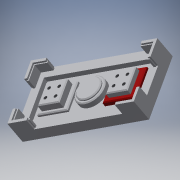
# Autodesk Inventor part: batteryCellTop
Saved by Autodesk Inventor 2019 (Build 230136000, 136)
## iProperties
Created: 2013-02-12
Part Number: batteryCellTop
Material: Aluminum 6061
Document SubType Name: Modeling
Designer: user
Density: 2.71 g/cm^3
Mass: 246.958 g
Surface Area: 283.047 cm^2
Volume: 91.1285 cm^3
Appearance: Aluminum - Flat
Description: BattTop
Author: user
Revision Number: 1
Autodesk Inventor part; units mm, degrees
ref_plane "YZ Plane" through (0, 0, 0) normal (1, 0, 0) x (0, 1, 0)
ref_plane "XZ Plane" through (0, 0, 0) normal (0, 1, 0) x (-1, 0, 0)
ref_plane "XY Plane" through (0, 0, 0) normal (0, 0, 1) x (1, 0, 0)
sketch "Sketch1" plane through (0, 0, 0) normal (0, 1, 0) x (-1, 0, 0)
  line L0 (62.25, -32.4) -> (-62.25, -32.4)
  line L1 (-62.25, -32.4) -> (-62.25, 32.4)
  line L2 (-62.25, 32.4) -> (62.25, 32.4)
  line L3 (62.25, 32.4) -> (62.25, -32.4)
  point P0 (0, 0)
  point P1 (62.25, 0)
  point P2 (0, -32.4)
  dimension "d0" = 64.8
  dimension "d2" = 124.5
  constraints: 8 end point, 2 midpoint, 2 parallel, 1 horizontal, 1 horizontal alignment, 1 perpendicular, 1 vertical alignment
  measures "d0" distance of L2.end L0.start
  measures "d2" distance of L0.start L0.end
extrude "Extrusion1" add sketch "Sketch1" along normal blind 11.45
sketch "Sketch2" plane through (0, 11.45, 0) normal (0, 1, 0) x (1, 0, 0)
  line L0 (62.25, 32.4) -> (-62.25, 32.4) projected
  line L1 (-62.25, 32.4) -> (-62.25, -32.4) projected
  line L2 (-62.25, -32.4) -> (62.25, -32.4) projected
  line L3 (62.25, -32.4) -> (62.25, 32.4) projected
  line L4 (-62.25, -13.55) -> (-62.25, -32.4)
  line L5 (-62.25, -32.4) -> (-46.85, -32.4)
  line L6 (-46.85, -32.4) -> (-46.85, -29.5)
  line L7 (-46.85, -29.5) -> (-59.35, -29.5)
  line L8 (-59.35, -29.5) -> (-59.35, -13.55)
  line L9 (-59.35, -13.55) -> (-62.25, -13.55)
  line L10 (62.25, -13.55) -> (59.35, -13.55)
  line L11 (59.35, -13.55) -> (59.35, -29.5)
  line L12 (59.35, -29.5) -> (46.85, -29.5)
  line L13 (46.85, -29.5) -> (46.85, -32.4)
  line L14 (62.25, -32.4) -> (62.25, -13.55)
  line L15 (46.85, -32.4) -> (62.25, -32.4)
  line L16 (43.4, 32.4) -> (43.4, 29.5)
  line L17 (43.4, 29.5) -> (59.35, 29.5)
  line L18 (62.25, 32.4) -> (43.4, 32.4)
  line L19 (59.35, 29.5) -> (59.35, 17)
  line L20 (59.35, 17) -> (62.25, 17)
  line L21 (62.25, 17) -> (62.25, 32.4)
  line L22 (-62.25, 17) -> (-59.35, 17)
  line L23 (-59.35, 17) -> (-59.35, 29.5)
  line L24 (-59.35, 29.5) -> (-43.4, 29.5)
  line L25 (-43.4, 29.5) -> (-43.4, 32.4)
  line L26 (-62.25, 32.4) -> (-62.25, 17)
  line L27 (-43.4, 32.4) -> (-62.25, 32.4)
  point P0 (0, 0)
  dimension "d5" = 18.85
  dimension "d7" = 15.4
  dimension "d8" = 2.9
  dimension "d9" = 2.9
  dimension "d10" = 18.85
  dimension "d11" = 2.9
  dimension "d12" = 2.9
  dimension "d13" = 15.4
  dimension "d21" = 15.4
  dimension "d22" = 18.85
  dimension "d23" = 2.9
  dimension "d24" = 2.9
  dimension "d28" = 15.4
  dimension "d29" = 2.9
  dimension "d30" = 2.9
  dimension "d31" = 18.85
  constraints: 48 end point, 13 parallel, 9 perpendicular, 6 collinear, 2 point on line
  measures "d5" distance between parallel lines of L5 L9
  measures "d7" distance of L4.end L5.end
  measures "d8" distance between parallel lines of L8 L4
  measures "d9" distance between parallel lines of L5 L7
  measures "d10" distance of L2.end L10.start
  measures "d11" distance of L10.start L10.end
  measures "d12" distance of L12.end L13.end
  measures "d13" distance of L13.end L2.end
  measures "d21" distance between parallel lines of L18 L20
  measures "d22" distance of L18.start L18.end
  measures "d23" distance between parallel lines of L19 L21
  measures "d24" distance between parallel lines of L18 L17
  measures "d28" distance of L27.end L26.end
  measures "d29" distance of L26.end L23.start
  measures "d30" distance of L24.end L27.start
  measures "d31" distance of L27.start L27.end
extrude "Extrusion2" add sketch "Sketch2" along normal blind 11.3 contours L3 L20 L19 L17 L16 L0 | L25 L24 L23 L22 L1 L0 | L3 L2 L13 L12 L11 L10 | L9 L8 L7 L6 L2 L1
sketch "Sketch3" plane through (0, 11.45, 0) normal (0, 1, 0) x (1, 0, 0)
  line L0 (43.4, 32.4) -> (-43.4, 32.4) projected
  line L1 (-62.25, 17) -> (-62.25, -13.55) projected
  line L2 (-46.85, -32.4) -> (46.85, -32.4) projected
  line L3 (62.25, -13.55) -> (62.25, 17) projected
  line L4 (-53.25, 22.4) -> (53.25, 22.4)
  line L5 (53.25, 22.4) -> (53.25, -22.4)
  line L6 (53.25, -22.4) -> (-53.25, -22.4)
  line L7 (-53.25, -22.4) -> (-53.25, 22.4)
  point P0 (0, 0)
  dimension "d41" = 9
  dimension "d42" = 9
  dimension "d43" = 10
  dimension "d44" = 10
  constraints: 8 end point, 2 parallel, 1 horizontal, 1 perpendicular
  measures "d41" distance between parallel lines of L1 L7
  measures "d42" distance between parallel lines of L3 L5
  measures "d43" distance between parallel lines of L4 L0
  measures "d44" distance between parallel lines of L2 L6
extrude "Extrusion3" cut sketch "Sketch3" against normal blind 5.1
sketch "Sketch4" plane through (0, 6.35, 0) normal (0, 1, 0) x (1, 0, 0)
  line L0 (-53.25, -22.4) -> (-53.25, 22.4) projected
  line L1 (-49.65, 15.75) -> (-17.15, 15.75)
  line L2 (-17.15, 15.75) -> (-17.15, -15.75)
  line L3 (-17.15, -15.75) -> (-49.65, -15.75)
  line L4 (-49.65, -15.75) -> (-49.65, 15.75)
  line L5 (43.4, 32.4) -> (-43.4, 32.4) projected
  point P0 (0, 0)
  dimension "d47" = 32.5
  dimension "d49" = 31.5
  dimension "d50" = 16.65
  dimension "d51" = 3.6
  constraints: 8 end point, 2 parallel, 1 horizontal, 1 perpendicular
  measures "d47" distance between parallel lines of L2 L4
  measures "d49" distance between parallel lines of L3 L1
  measures "d50" distance between parallel lines of L1 L5
  measures "d51" distance between parallel lines of L4 L0
extrude "Extrusion4" add sketch "Sketch4" along normal blind 4.6
sketch "Sketch5" plane through (0, 10.95, 0) normal (0, 1, 0) x (1, 0, 0)
  line L0 (-17.15, 15.75) -> (-49.65, 15.75) projected
  line L1 (-49.65, 15.75) -> (-49.65, -15.75) projected
  line L2 (-44.1, 11.95) -> (-22.7, 11.95)
  line L3 (-22.7, 11.95) -> (-22.7, -11.95)
  line L4 (-22.7, -11.95) -> (-44.1, -11.95)
  line L5 (-44.1, -11.95) -> (-44.1, 11.95)
  point P0 (0, 0)
  point P1 (-33.4, 11.95)
  point P2 (-33.4, 15.75)
  point P3 (-44.1, 0)
  point P4 (-49.65, 0)
  dimension "d54" = 21.4
  dimension "d56" = 23.9
  constraints: 8 end point, 4 midpoint, 2 parallel, 1 horizontal, 1 horizontal alignment, 1 perpendicular, 1 vertical alignment
  measures "d54" distance of L2.start L2.end
  measures "d56" distance between parallel lines of L4 L2
extrude "Extrusion5" add sketch "Sketch5" along normal blind 5.5
sketch "Sketch6" plane through (0, 6.35, 0) normal (0, 1, 0) x (1, 0, 0)
  line L0 (53.25, 22.4) -> (53.25, -22.4) projected
  line L1 (18.73, 14.8) -> (48.73, 14.8)
  line L2 (48.73, 14.8) -> (48.73, -14.8)
  line L3 (48.73, -14.8) -> (18.73, -14.8)
  line L4 (18.73, -14.8) -> (18.73, 14.8)
  point P0 (0, 0)
  point P1 (18.73, 0)
  dimension "d59" = 29.6
  dimension "d61" = 30
  dimension "d62" = 4.52
  constraints: 8 end point, 2 parallel, 1 horizontal, 1 horizontal alignment, 1 midpoint, 1 perpendicular
  measures "d59" distance between parallel lines of L3 L1
  measures "d61" distance of L1.start L1.end
  measures "d62" distance between parallel lines of L0 L2
extrude "Extrusion6" add sketch "Sketch6" along normal blind 2.8
sketch "Sketch7" plane through (0, 9.15, 0) normal (0, 1, 0) x (1, 0, 0)
  line L0 (48.73, 14.8) -> (18.73, 14.8) projected
  line L1 (18.73, 14.8) -> (18.73, -14.8) projected
  line L2 (23.03, 11.95) -> (44.43, 11.95)
  line L3 (44.43, 11.95) -> (44.43, -11.95)
  line L4 (44.43, -11.95) -> (23.03, -11.95)
  line L5 (23.03, -11.95) -> (23.03, 11.95)
  point P0 (0, 0)
  point P1 (23.03, 0)
  point P2 (18.73, 0)
  point P3 (33.73, 11.95)
  point P4 (33.73, 14.8)
  dimension "d65" = 21.4
  dimension "d67" = 23.9
  constraints: 8 end point, 4 midpoint, 2 parallel, 1 horizontal, 1 horizontal alignment, 1 perpendicular, 1 vertical alignment
  measures "d65" distance of L2.start L2.end
  measures "d67" distance of L2.end L3.end
extrude "Extrusion7" add sketch "Sketch7" along normal blind 7.3
sketch "Sketch8" plane through (0, 11.45, 0) normal (0, 1, 0) x (1, 0, 0)
  line L0 (62.25, -13.55) -> (62.25, 17) projected
  line L1 (-60.55, -12.55) -> (-60.55, -13.55)
  line L2 (-60.55, -13.55) -> (-59.35, -13.55)
  line L3 (-59.35, -13.55) -> (-59.35, -29.5)
  line L4 (-59.35, -29.5) -> (-46.85, -29.5)
  line L5 (-46.85, -29.5) -> (-46.85, -30.7)
  line L6 (-46.85, -30.7) -> (-45.85, -30.7)
  line L7 (-45.85, -30.7) -> (-45.85, -28.5)
  line L8 (-45.85, -28.5) -> (-58.35, -28.5)
  line L9 (-58.35, -28.5) -> (-58.35, -12.55)
  line L10 (-58.35, -12.55) -> (-60.55, -12.55)
  line L11 (-59.35, -13.55) -> (-62.25, -13.55) projected
  line L12 (-59.35, -29.5) -> (-59.35, -13.55) projected
  line L13 (-46.85, -29.5) -> (-59.35, -29.5) projected
  line L14 (-46.85, -32.4) -> (-46.85, -29.5) projected
  line L15 (60.55, 16) -> (60.55, 17)
  line L16 (60.55, 17) -> (59.35, 17)
  line L17 (59.35, 17) -> (59.35, 29.5)
  line L18 (59.35, 29.5) -> (43.4, 29.5)
  line L19 (43.4, 29.5) -> (43.4, 30.7)
  line L20 (43.4, 30.7) -> (42.4, 30.7)
  line L21 (42.4, 30.7) -> (42.4, 28.5)
  line L22 (42.4, 28.5) -> (58.35, 28.5)
  line L23 (58.35, 28.5) -> (58.35, 16)
  line L24 (58.35, 16) -> (60.55, 16)
  line L25 (43.4, 29.5) -> (59.35, 29.5) projected
  line L26 (59.35, 29.5) -> (59.35, 17) projected
  line L27 (59.35, 17) -> (62.25, 17) projected
  line L28 (43.4, 32.4) -> (43.4, 29.5) projected
  line L29 (-60.55, 16) -> (-58.35, 16)
  line L30 (-58.35, 16) -> (-58.35, 28.5)
  line L31 (-58.35, 28.5) -> (-42.4, 28.5)
  line L32 (-42.4, 28.5) -> (-42.4, 30.7)
  line L33 (-42.4, 30.7) -> (-43.4, 30.7)
  line L34 (-43.4, 30.7) -> (-43.4, 29.5)
  line L35 (-43.4, 29.5) -> (-59.35, 29.5)
  line L36 (-59.35, 29.5) -> (-59.35, 17)
  line L37 (-59.35, 17) -> (-60.55, 17)
  line L38 (-60.55, 17) -> (-60.55, 16)
  line L39 (-59.35, 29.5) -> (-43.4, 29.5) projected
  line L40 (-59.35, 17) -> (-59.35, 29.5) projected
  line L41 (-43.4, 29.5) -> (-43.4, 32.4) projected
  line L42 (-62.25, 17) -> (-59.35, 17) projected
  line L43 (60.55, -12.55) -> (58.35, -12.55)
  line L44 (58.35, -12.55) -> (58.35, -28.5)
  line L45 (58.35, -28.5) -> (45.85, -28.5)
  line L46 (45.85, -28.5) -> (45.85, -30.7)
  line L47 (45.85, -30.7) -> (46.85, -30.7)
  line L48 (46.85, -30.7) -> (46.85, -29.5)
  line L49 (46.85, -29.5) -> (59.35, -29.5)
  line L50 (59.35, -29.5) -> (59.35, -13.55)
  line L51 (59.35, -13.55) -> (60.55, -13.55)
  line L52 (60.55, -13.55) -> (60.55, -12.55)
  line L53 (59.35, -13.55) -> (59.35, -29.5) projected
  line L54 (62.25, -13.55) -> (59.35, -13.55) projected
  line L55 (59.35, -29.5) -> (46.85, -29.5) projected
  line L56 (46.85, -29.5) -> (46.85, -32.4) projected
  point P0 (0, 0)
  dimension "d70" = 1
  dimension "d72" = 1
  dimension "d73" = 1
  dimension "d74" = 1
  dimension "d76" = 2.2
  dimension "d77" = 2.2
  dimension "d78" = 1
  dimension "d79" = 1
  dimension "d80" = 1
  dimension "d81" = 1
  dimension "d82" = 2.2
  dimension "d83" = 2.2
  dimension "d86" = 2.2
  dimension "d87" = 1
  dimension "d88" = 1
  dimension "d89" = 1
  dimension "d90" = 1
  dimension "d91" = 2.2
  dimension "d92" = 2.2
  dimension "d93" = 1
  dimension "d94" = 1
  dimension "d95" = 1
  dimension "d96" = 1
  dimension "d97" = 2.2
  constraints: 80 end point, 33 parallel, 16 collinear, 4 perpendicular
  measures "d70" distance between parallel lines of L2 L10
  measures "d72" distance of L5.end L6.end
  measures "d73" distance between parallel lines of L4 L8
  measures "d74" distance between parallel lines of L9 L3
  measures "d76" distance of L9.end L1.start
  measures "d77" distance of L6.end L7.end
  measures "d78" distance between parallel lines of L16 L24
  measures "d79" distance of L19.end L20.end
  measures "d80" distance between parallel lines of L18 L22
  measures "d81" distance between parallel lines of L23 L17
  measures "d82" distance of L24.start L24.end
  measures "d83" distance of L20.end L22.start
  measures "d86" distance of L29.start L29.end
  measures "d87" distance of L37.end L29.start
  measures "d88" distance of L32.end L33.end
  measures "d89" distance between parallel lines of L30 L36
  measures "d90" distance between parallel lines of L35 L31
  measures "d91" distance of L31.end L32.end
  measures "d92" distance of L52.end L44.start
  measures "d93" distance of L51.end L52.end
  measures "d94" distance of L47.start L48.start
  measures "d95" distance between parallel lines of L44 L50
  measures "d96" distance between parallel lines of L49 L45
  measures "d97" distance of L45.end L47.start
extrude "Extrusion8" add sketch "Sketch8" along normal blind 9.5
sketch "Sketch10" plane through (0, 6.35, 0) normal (0, 1, 0) x (1, 0, 0)
  circle A0 centre (0, 0) radius 14.5
  dimension "d133" = 29
  constraints: 1 centre point
  measures "d133" diameter of A0
extrude "Extrusion10" add sketch "Sketch10" along normal blind 6
sketch "Sketch11" plane through (0, 12.35, 0) normal (0, 1, 0) x (1, 0, 0)
  circle A0 centre (0, 0) radius 12
  dimension "d137" = 24
  constraints: 1 centre point
  measures "d137" diameter of A0
extrude "Extrusion11" add sketch "Sketch11" along normal blind 2
chamfer "Chamfer1" distance 1 angle 45 4 edges at (44.43, 16.45, 0) (33.73, 16.45, 11.95) (23.03, 16.45, 0) (33.73, 16.45, -11.95)
chamfer "Chamfer2" distance 1 angle 45 4 edges at (-33.4, 16.45, -11.95) (-44.1, 16.45, 0) (-33.4, 16.45, 11.95) (-22.7, 16.45, 0)
chamfer "Chamfer3" distance 1 angle 45 4 edges at (-33.4, 10.95, 15.75) (-49.65, 10.95, 0) (-33.4, 10.95, -15.75) (-17.15, 10.95, 0)
chamfer "Chamfer4" distance 1 angle 45 4 edges at (33.73, 9.15, -14.8) (18.73, 9.15, 0) (33.73, 9.15, 14.8) (48.73, 9.15, 0)
sketch "Sketch12" plane through (0, 16.45, 0) normal (0, 1, 0) x (1, 0, 0)
  line L0 (23.03, 11.95) -> (23.03, -11.95) projected
  point P0 (0, 0)
  point P1 (38.73, -5)
  point P2 (28.73, -5)
  point P3 (28.73, 5)
  point P4 (38.73, 5)
  point P5 (-38.1211, 5.7215)
  point P6 (-28.8217, 5.7215)
  point P7 (-28.8217, -4.174)
  point P8 (-38.1211, -5)
  dimension "d153" = 10
  dimension "d155" = 10
  dimension "d157" = 5
  dimension "d159" = 5.7
  constraints: 2 horizontal alignment, 2 vertical alignment
  measures "d153" distance of point (38.73, 5) point (28.73, 5)
  measures "d155" distance of point (28.73, -5) point (28.73, 5)
  measures "d157" vertical distance of point (0, 0) point (28.73, 5)
  measures "d159" distance from line of point (28.73, -5) L0
hole "Hole1" at (38.73, 16.45, 5) at (28.73, 16.45, 5) at (28.73, 16.45, -5) at (38.73, 16.45, -5) direction (0, -1, 0) diameter 3.459 depth 7 tip angle 118 thread size "M4x0.5" class "6H" standard "ISO Metric profile"
sketch "Sketch14" plane through (0, 16.45, 0) normal (0, 1, 0) x (1, 0, 0)
  line L0 (-44.1, 11.95) -> (-44.1, -11.95) projected
  point P0 (0, 0)
  point P1 (-38.4, 5)
  point P2 (-28.4, 5)
  point P3 (-28.4, -5)
  point P4 (-38.4, -5)
  dimension "d167" = 10
  dimension "d169" = 10
  dimension "d170" = 5
  dimension "d171" = 5.7
  constraints: 2 horizontal alignment, 2 vertical alignment
  measures "d167" distance of point (-28.4, 5) point (-38.4, 5)
  measures "d169" distance of point (-38.4, -5) point (-38.4, 5)
  measures "d170" vertical distance of point (0, 0) point (-28.4, 5)
  measures "d171" distance from line of L0 point (-38.4, 5)
hole "Hole2" at (-38.4, 16.45, -5) at (-28.4, 16.45, -5) at (-28.4, 16.45, 5) at (-38.4, 16.45, 5) direction (0, -1, 0) diameter 3.459 depth 7 tip angle 118 thread size "M4x0.5" class "6H" standard "ISO Metric profile"
chamfer "Chamfer5" distance 1 angle 45 2 edges at (-12, 14.35, 0) (-14.5, 12.35, 0)
equation "\"d0\" = BtDp"
equation "\"d2\" = BtWd"
equation "\"d3\" = ModHt"
equation "\"d5\" = TopOutSh"
equation "\"d7\" = TopOutLn"
equation "\"d8\" = TopOutDp"
equation "\"d9\" = d8"
equation "\"d10\" = d5"
equation "\"d11\" = d9"
equation "\"d12\" = d9"
equation "\"d13\" = d7"
equation "\"d21\" = d25"
equation "\"d22\" = d26"
equation "\"d23\" = d27"
equation "\"d24\" = d23"
equation "\"d28\" = d32"
equation "\"d29\" = d33"
equation "\"d30\" = d33"
equation "\"d31\" = d34"
equation "\"d39\" = TopHoldHt"
equation "\"d41\" = LedgeSh"
equation "\"d42\" = d41"
equation "\"d43\" = LedgeLn"
equation "\"d44\" = d43"
equation "\"d45\" = InPdDp"
equation "\"d47\" = RedLeadPedesWd"
equation "\"d49\" = RedLeadPedesDp"
equation "\"d50\" = 0.5 * BtDp - 0.5 * RedLeadPedesDp"
equation "\"d51\" = RedLeadPedesGap"
equation "\"d52\" = RedLeadPedesHt"
equation "\"d54\" = RedLeadWd"
equation "\"d56\" = RedLeadDp"
equation "\"d57\" = RedLeadHt"
equation "\"d59\" = CyanLeadPedesWd"
equation "\"d61\" = CyanLeadPedesDp"
equation "\"d62\" = CyanLeadPedesGap"
equation "\"d63\" = CyanLeadPedesHt"
equation "\"d65\" = CyanLeadWd"
equation "\"d67\" = CyanLeadDp"
equation "\"d68\" = CyanLeadHt"
equation "\"d70\" = InCapHldWd"
equation "\"d72\" = d70"
equation "\"d73\" = d70"
equation "\"d74\" = d73"
equation "\"d76\" = InCapHldDp"
equation "\"d77\" = d76"
equation "\"d78\" = d84"
equation "\"d79\" = d78"
equation "\"d80\" = d78"
equation "\"d81\" = d80"
equation "\"d82\" = d85"
equation "\"d83\" = d82"
equation "\"d32\" = d35"
equation "\"d33\" = d36"
equation "\"d34\" = d37"
equation "\"d36\" = d38"
equation "\"BtDp\" = 64.8"
equation "\"BtWd\" = 124.5"
equation "\"ModHt\" = 11.45"
equation "\"TopOutSh\" = 18.85"
equation "\"TopOutLn\" = 15.4"
equation "\"TopOutDp\" = 2.9"
equation "\"d25\" = 15.4"
equation "\"d26\" = 18.85"
equation "\"d27\" = 2.9"
equation "\"TopHoldHt\" = 11.3"
equation "\"LedgeSh\" = 9"
equation "\"LedgeLn\" = 10"
equation "\"InPdDp\" = 5.1"
equation "\"RedLeadPedesWd\" = 32.5"
equation "\"RedLeadPedesDp\" = 31.5"
equation "\"RedLeadPedesGap\" = 3.6"
equation "\"RedLeadPedesHt\" = 4.6"
equation "\"RedLeadWd\" = 21.4"
equation "\"RedLeadDp\" = 23.9"
equation "\"RedLeadHt\" = 5.5"
equation "\"CyanLeadPedesWd\" = 29.6"
equation "\"CyanLeadPedesDp\" = 30"
equation "\"CyanLeadPedesGap\" = 4.52"
equation "\"CyanLeadPedesHt\" = 2.8"
equation "\"CyanLeadWd\" = 21.4"
equation "\"CyanLeadDp\" = 23.9"
equation "\"CyanLeadHt\" = 7.3"
equation "\"InCapHldWd\" = 1"
equation "\"InCapHldDp\" = 2.2"
equation "\"d84\" = 1"
equation "\"d85\" = 2.2"
equation "\"d35\" = 15.4"
equation "\"d37\" = 18.85"
equation "\"d38\" = 2.9"
body "Solid1"
